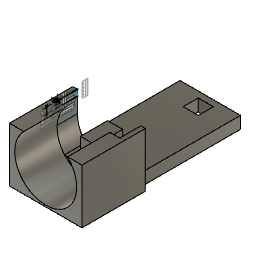
Toggle Box Base v3 (Autodesk Fusion 360 design; units mm, degrees)
Autodesk Fusion 360 part; units mm, degrees
note: some values were not read from the file. Chosen so that the rebuilt part matches the saved one: which face or edge a step refers to; which pieces of a blend or face edit are solid. Set by a fixed rule: which sketch regions a step uses.
sketch "Sketch1" plane through (0, 0, 0) normal (0, 0, 1) x (1, 0, 0)
  line L0 (0, 0) -> (16, 0)
  line L1 (16, 0) -> (16, 29.5)
  line L2 (16, 29.5) -> (0, 29.5)
  line L3 (0, 29.5) -> (0, 0)
  line L4 (-2, -2) -> (18, -2)
  line L5 (18, -2) -> (18, 31.5)
  line L6 (18, 31.5) -> (-2, 31.5)
  line L7 (-2, 31.5) -> (-2, -2)
  dimension "d1" = 16
  dimension "d2" = 29.5
  dimension "d3" = 2
  constraint horizontal L0
  constraint vertical L1
  constraint horizontal L2
  constraint vertical L3
  constraint coincident L0.start L3.end
  measures "d1" distance of L0.start L0.end
  measures "d2" distance of L0.start L2.end
extrude "Extrude1" add sketch "Sketch1" along normal blind 17 makes body 1
sketch "Sketch2" plane through (0, -2, 0) normal (0, -1, 0) x (1, 0, 0)
  line L0 (-2, 0) -> (18, 0)
  line L1 (18, 0) -> (18, 17)
  line L2 (18, 17) -> (-2, 17)
  line L3 (-2, 17) -> (-2, 0)
  line L4 (18, 17) -> (18, 9) construction
  line L5 (18, 9) -> (-2, 9) construction
  line L6 (8, 17) -> (5.5, 17) construction
  line L7 (5.5, 9) -> (2, 7) construction
  line L8 (5.5, 9) -> (10.5, 9) construction
  line L9 (10.5, 9) -> (10.5, 13) construction
  line L10 (10.5, 13) -> (5.5, 13) construction
  line L11 (5.5, 13) -> (5.5, 9) construction
  line L12 (5.5, 13) -> (10.5, 13)
  line L13 (10.5, 13) -> (10.5, 9)
  line L14 (10.5, 9) -> (5.5, 9)
  line L15 (5.5, 9) -> (5.5, 13)
  dimension "d6" = 8
  dimension "d7" = 2.5
  dimension "d8" = 5
  dimension "d9" = 4
  constraint coincident L1.end L2.start
  constraint perpendicular L2 L4
  constraint coincident L3 L5.end
  constraint perpendicular L3 L5
  constraint midpoint L2 L6.start
  constraint coincident L2 L6.end
  constraint coincident L5 L7.start
  constraint horizontal L8
  constraint vertical L9
  constraint horizontal L10
  constraint vertical L11
  constraint horizontal L12
  constraint vertical L13
  constraint horizontal L14
  constraint vertical L15
  measures "d6" distance of L1.end L4.end
  measures "d7" distance of L6.start L6.end
  measures "d8" distance of L7.start L8.end
  measures "d9" distance of L7.start L10.end
extrude "Extrude2" cut sketch "Sketch2" against normal blind 11 contours L12 L13 L14 L15 bodies 1
extrude "Extrude3" add 1 faces at (-1.3333, 19.6667, 0) along direction (0, 0, -1) blind 2 on bodies 1 bodies 1
sketch "Sketch3" plane through (18, 0, 0) normal (1, 0, 0) x (0, 1, 0)
  line L0 (31.5, -2) -> (31.5, 17)
  line L1 (31.5, 17) -> (-2, 17)
  line L2 (-2, 17) -> (-2, -2)
  line L3 (-2, -2) -> (31.5, -2)
  line L4 (-2, -2) -> (31.5, -2)
  line L5 (31.5, -2) -> (31.5, 0)
  line L6 (31.5, 0) -> (-2, 0)
  line L7 (-2, 0) -> (-2, -2)
  dimension "d14" = 2
  constraint horizontal L4
  constraint vertical L5
  constraint horizontal L6
  constraint vertical L7
  constraint coincident L2.end L3.start
  measures "d14" distance of L2.end L6.end
extrude "Extrude4" add sketch "Sketch3" against normal blind 18 contours L0 L2 L3 L4 L5 L6 L7 bodies 1
sketch "Sketch4" plane through (0, 0, 0) normal (0, 0, 1) x (-1, 0, 0)
  line L0 (-16, -29.5) -> (0, -29.5)
  line L1 (0, -29.5) -> (0, 0)
  line L2 (0, 0) -> (-16, 0)
  line L3 (-16, 0) -> (-16, -29.5)
  line L4 (-8, -29.5) -> (-5, -29.5) construction
  line L5 (-5, -29.5) -> (-11, -29.5)
  line L6 (-11, -29.5) -> (-11, -24.5)
  line L7 (-11, -24.5) -> (-5, -24.5)
  line L8 (-5, -24.5) -> (-5, -29.5)
  line L9 (-11, 0) -> (-5, 0)
  line L10 (-5, 0) -> (-5, -5)
  line L11 (-5, -5) -> (-11, -5)
  line L12 (-11, -5) -> (-11, 0)
  dimension "d17" = 3
  dimension "d18" = 6
  dimension "d19" = 5
  dimension "d20" = 6
  dimension "d21" = 5
  constraint midpoint L0 L4.start
  constraint parallel L0 L4
  constraint horizontal L5
  constraint vertical L6
  constraint horizontal L7
  constraint vertical L8
  constraint horizontal L9
  constraint vertical L10
  constraint horizontal L11
  constraint vertical L12
  constraint coincident L2 L9.start
  measures "d17" distance of L4.start L4.end
  measures "d18" distance of L4.end L5.end
  measures "d19" distance of L4.end L7.end
  measures "d20" distance of L9.start L9.end
  measures "d21" distance of L9.start L11.end
extrude "Extrude5" cut sketch "Sketch4" against normal blind 14 contours L0 L5 L6 L7 L8 | L2 L9 L10 L11 L12 bodies 1
extrude "Extrude6" cut 1 faces at (0.3333, 18, -2) along direction (0, 0, 1) blind 2 on bodies 1 bodies 1
extrude "Extrude7" cut 1 faces at (8.8333, -1.3333, 9) along direction (0, 0, -1) blind 25 on bodies 1 bodies 1
extrude "Extrude8" add 1 faces at (-1.3333, 19.6667, 17) along direction (0, 0, 1) blind 1 on bodies 1 bodies 1
sketch "Sketch5" plane through (0, 31.5, 0) normal (0, 1, 0) x (-1, 0, 0)
  line L0 (-18, 0) -> (2, 0)
  line L1 (2, 0) -> (2, 18)
  line L2 (2, 18) -> (-18, 18)
  line L3 (-18, 18) -> (-18, 0)
  line L4 (-18, 18) -> (2, 18)
  line L5 (2, 18) -> (2, 17)
  line L6 (2, 17) -> (-18, 17)
  line L7 (-18, 17) -> (-18, 18)
  dimension "d30" = 1
  constraint horizontal L4
  constraint vertical L5
  constraint horizontal L6
  constraint vertical L7
  constraint coincident L1 L5.end
  constraint coincident L2.end L3.start
  measures "d30" distance of L2.end L6.end
extrude "Extrude9" add sketch "Sketch5" against normal blind 31.5 contours L1 L2 L3 L4 L5 L6 L7 bodies 1
sketch "Sketch6" plane through (0, 0, 18) normal (0, 0, 1) x (-1, 0, 0)
  line L0 (2, -31.5) -> (2, 2)
  line L1 (2, 2) -> (-18, 2)
  line L2 (-18, 2) -> (-18, -31.5)
  line L3 (-18, -31.5) -> (2, -31.5)
  line L4 (2, -31.5) -> (-18, 2) construction
  circle A0 centre (-8, -14.75) radius 6.25
  dimension "d33" = 12.5
  constraint coincident L0.start L3.end
  constraint coincident L1.end L2.start
  constraint midpoint L4 A0.centre
  measures "d33" diameter of A0
extrude "Extrude10" cut sketch "Sketch6" against normal blind 6 contours A0 bodies 1
extrude "Extrude11" add 1 faces at (-1.3333, 19.6667, 0) along direction (0, 0, -1) blind 2 on bodies 1 bodies 1
extrude "Extrude12" cut 1 faces at (7.8443, 27.9942, 18) along direction (0, 0, -1) blind 18 on bodies 1 bodies 1
sketch "Sketch7" plane through (0, 0, 0) normal (0, 0, 1) x (-1, 0, 0)
  line L0 (-5.5, 2) -> (-5.5, 0)
  line L1 (-5.5, 0) -> (0, 0)
  line L2 (0, 0) -> (0, -29.5)
  line L3 (0, -29.5) -> (-16, -29.5)
  line L4 (-16, -29.5) -> (-16, 0)
  line L5 (-16, 0) -> (-10.5, 0)
  line L6 (-10.5, 0) -> (-10.5, 2)
  line L7 (-10.5, 2) -> (-18, 2)
  line L8 (-18, 2) -> (-18, -31.5)
  line L9 (-18, -31.5) -> (2, -31.5)
  line L10 (2, -31.5) -> (2, 2)
  line L11 (2, 2) -> (-5.5, 2)
  line L12 (-5.5, 0) -> (-10.5, 0)
  line L13 (-10.5, 0) -> (-10.5, 2)
  line L14 (-10.5, 2) -> (-5.5, 2)
  line L15 (-5.5, 2) -> (-5.5, 0)
  constraint horizontal L12
  constraint vertical L13
  constraint horizontal L14
  constraint vertical L15
  constraint coincident L6.end L7.start
  constraint coincident L0.end L1.start
extrude "Extrude13" add sketch "Sketch7" along normal blind 8 separate body contours L0 L6 L12 L13 L14 L15 makes body 2
extrude "Extrude14" add 1 faces at (5.5, -1.3333, -0.6667) along direction (1, 0, 0) blind 6 on bodies 1 bodies 1 2
sketch "Sketch8" plane through (0, 0, -2) normal (0, 0, -1) x (1, 0, 0)
  line L0 (0, 0) -> (16, 0)
  line L1 (16, 0) -> (16, -29.5)
  line L2 (16, -29.5) -> (0, -29.5)
  line L3 (0, -29.5) -> (0, 0)
  line L4 (18, 2) -> (-2, 2)
  line L5 (-2, 2) -> (-2, -31.5)
  line L6 (-2, -31.5) -> (18, -31.5)
  line L7 (18, -31.5) -> (18, 2)
extrude "Extrude15" add sketch "Sketch8" against normal blind 2 contours L0 L1 L2 L3 bodies 1
sketch "Sketch9" plane through (0, -2, 0) normal (0, -1, 0) x (1, 0, 0)
  line L0 (-2, -2) -> (18, -2)
  line L1 (18, -2) -> (18, 0)
  line L2 (18, 0) -> (10.5, 0)
  line L3 (10.5, 0) -> (10.5, 8)
  line L4 (10.5, 8) -> (5.5, 8)
  line L5 (5.5, 8) -> (5.5, 0)
  line L6 (5.5, 0) -> (-2, 0)
  line L7 (-2, 0) -> (-2, -2)
  line L8 (5.5, 0) -> (10.5, 0)
  constraint coincident L5.end L6.start
  constraint coincident L2.end L3.start
extrude "Extrude16" add sketch "Sketch9" along normal blind 6 contours L0 L1 L2 L6 L7 L8 bodies 1
sketch "Sketch10" plane through (0, 0, 0) normal (0, 0, 1) x (-1, 0, 0)
  line L0 (-18, 8) -> (-18, -31.5)
  line L1 (-18, -31.5) -> (2, -31.5)
  line L2 (2, -31.5) -> (2, 8)
  line L3 (2, 8) -> (-18, 8)
  line L4 (-10.5, 2) -> (-5.5, 2)
  line L5 (-5.5, 2) -> (-5.5, 0)
  line L6 (-5.5, 0) -> (-10.5, 0)
  line L7 (-10.5, 0) -> (-10.5, 2)
  line L8 (2, 8) -> (-18, 8)
  line L9 (-18, 8) -> (-18, 2)
  line L10 (-18, 2) -> (2, 2)
  line L11 (2, 2) -> (2, 8)
  constraint horizontal L8
  constraint vertical L9
  constraint horizontal L10
  constraint vertical L11
  constraint coincident L0 L9.end
  constraint coincident L2.end L3.start
extrude "Extrude17" add sketch "Sketch10" along normal blind 18 contours L0 L2 L3 L4 L8 L9 L10 L11 bodies 1
sketch "Sketch11" plane through (0, -8, 0) normal (0, -1, 0) x (1, 0, 0)
  line L0 (-2, 18) -> (-2, -2)
  line L1 (-2, -2) -> (18, -2)
  line L2 (18, -2) -> (18, 18)
  line L3 (18, 18) -> (-2, 18)
  line L4 (8, 18) -> (8, 7) construction
  circle A0 centre (8, 7) radius 10
  dimension "d50" = 11
  dimension "d51" = 20
  constraint midpoint L3 L4.start
  constraint perpendicular L3 L4
  constraint coincident L4.end A0.centre
  measures "d50" distance of L4.start L4.end
  measures "d51" diameter of A0
extrude "Extrude18" add 1 faces at (7.1667, -6, 18) along direction (0, 0, -1) blind 22 on bodies 1 bodies 1
extrude "Extrude19" cut sketch "Sketch11" against normal blind 6 contours L1 A0 | L1 A0 bodies 1
extrude "Extrude20" add 2 faces at (0.1449, -8, 15.54) (0.1449, -8, -1.54) along direction (0, -1, 0) blind 15 on bodies 1 bodies 1
extrude "Extrude21" cut 1 faces at (-2, -9, 10.6667) along direction (1, 0, 0) blind 37 on bodies 1 bodies 1
extrude "Extrude22" add 1 faces at (8.8333, -2, 5.3333) along direction (0, -1, 0) blind 7 on bodies 1 bodies 1
sketch "Sketch12" plane through (0, 0, -2) normal (0, 0, -1) x (1, 0, 0)
  line L0 (18, 2) -> (12.3589, 2)
  line L1 (12.3589, 2) -> (12.3589, 9)
  line L2 (12.3589, 9) -> (3.6411, 9)
  line L3 (3.6411, 9) -> (3.6411, 2)
  line L4 (3.6411, 2) -> (-2, 2)
  line L5 (-2, 2) -> (-2, -31.5)
  line L6 (-2, -31.5) -> (18, -31.5)
  line L7 (18, -31.5) -> (18, 2)
  line L8 (12.3589, 2) -> (3.6411, 2)
  constraint coincident L0.end L1.start
  constraint coincident L3.end L4.start
extrude "Extrude23" add sketch "Sketch12" along normal blind 2 contours L1 L2 L3 L8 bodies 1
sketch "Sketch13" plane through (-2, 0, 0) normal (-1, 0, 0) x (0, -1, 0)
  line L0 (23, 7) -> (2, 7)
  line L1 (2, 7) -> (2, 0)
  line L2 (2, 0) -> (-31.5, 0)
  line L3 (-31.5, 0) -> (-31.5, -2)
  line L4 (-31.5, -2) -> (2, -2)
  line L5 (2, -2) -> (2, -4)
  line L6 (2, -4) -> (23, -4)
  line L7 (23, -4) -> (23, 7)
  line L8 (2, 0) -> (2, -2)
  constraint coincident L1.end L2.start
  constraint coincident L4.end L5.start
extrude "Extrude24" add sketch "Sketch13" along normal blind 2 contours L0 L1 L5 L6 L7 L8 bodies 1
sketch "Sketch14" plane through (18, 0, 0) normal (1, 0, 0) x (0, 1, 0)
  line L0 (-2, 7) -> (-23, 7)
  line L1 (-23, 7) -> (-23, -4)
  line L2 (-23, -4) -> (-2, -4)
  line L3 (-2, -4) -> (-2, -2)
  line L4 (-2, -2) -> (31.5, -2)
  line L5 (31.5, -2) -> (31.5, 0)
  line L6 (31.5, 0) -> (-2, 0)
  line L7 (-2, 0) -> (-2, 7)
  line L8 (-2, 0) -> (-2, -2)
  constraint coincident L6.end L7.start
  constraint coincident L3.end L4.start
extrude "Extrude25" add sketch "Sketch14" along normal blind 2 contours L0 L1 L2 L3 L7 L8 bodies 1
extrude "Extrude26" add 2 faces at (19.3333, -9, 7) (-2.6667, -9, 7) along direction (0, 0, 1) blind 7 on bodies 1 bodies 1
move_face "OffsetFaces1" offset -0.5 3 faces at (18, -16, 11.6667) (16.6713, -16, 2.0193) (-2, -9, 9.3333) on bodies 1
sketch "Sketch15" plane through (0, -23, 0) normal (0, -1, 0) x (1, 0, 0)
  arc A0 (-2.5, 7) -> (18.5, 7) centre (8, 7) ccw
  line L0 (-2.5, 7) -> (-2.5, 14)
  line L1 (-2.5, 14) -> (-4, 14)
  line L2 (-4, 14) -> (-4, -4)
  line L3 (-4, -4) -> (20, -4)
  line L4 (20, -4) -> (20, 14)
  line L5 (20, 14) -> (18.5, 14)
  line L6 (18.5, 14) -> (18.5, 7)
  line L7 (8, -3.5) -> (8, -2.25) construction
  line L8 (8, -3.5) -> (8, 6.75) construction
  circle A1 centre (8, 6.75) radius 10.25
  line L9 (20, -4) -> (-4, -4)
  line L10 (-4, -4) -> (-4, 14)
  line L11 (-4, 14) -> (20, 14)
  line L12 (20, 14) -> (20, -4)
  dimension "d71" = 1.25
  dimension "d72" = 10.25
  constraint midpoint A0 L7.start
  constraint perpendicular L3 L7
  constraint parallel L7 L8
  constraint coincident L8.end A1.centre
  constraint coincident L7.start A1
  constraint horizontal L9
  constraint vertical L10
  constraint horizontal L11
  constraint vertical L12
  constraint coincident L1.end L2.start
  constraint coincident L3.end L4.start
  measures "d71" distance of L7.start L7.end
  measures "d72" distance of L7.start L8.end
extrude "Extrude27" add sketch "Sketch15" against normal blind 14 contours A0 L0 A1 L11 | A0 L6 A1 L11 bodies 1
sketch "Sketch16" plane through (-2.5, 0, 0) normal (1, 0, 0) x (0, 1, 0)
  line L0 (-9, 14) -> (-9, 7)
  line L1 (-9, 7) -> (-2, 7)
  line L2 (-2, 7) -> (-2, 14)
  line L3 (-2, 14) -> (-9, 14)
  line L4 (-9, 14) -> (-2, 14)
  line L5 (-2, 14) -> (-2, 12)
  line L6 (-2, 12) -> (-9, 12)
  line L7 (-9, 12) -> (-9, 14)
  dimension "d75" = 2
  constraint horizontal L4
  constraint vertical L5
  constraint horizontal L6
  constraint vertical L7
  constraint coincident L0.start L3.end
  measures "d75" distance of L0.start L6.end
sketch "Sketch17" plane through (0, 0, 0) normal (0, 0, 1) x (-1, 0, 0)
  line L0 (-15.8262, 2) -> (-18, 2)
  line L1 (-18, 2) -> (-18, -31.5)
  line L2 (-18, -31.5) -> (2, -31.5)
  line L3 (2, -31.5) -> (2, 2)
  line L4 (2, 2) -> (-0.1738, 2)
  line L5 (-0.1738, 2) -> (-0.1738, 9)
  line L6 (-0.1738, 9) -> (-0.2864, 9)
  line L7 (-0.2864, 9) -> (-5.5, 9)
  line L8 (-5.5, 9) -> (-5.5, 0)
  line L9 (-5.5, 0) -> (-10.5, 0)
  line L10 (-10.5, 0) -> (-10.5, 9)
  line L11 (-10.5, 9) -> (-15.7136, 9)
  line L12 (-15.7136, 9) -> (-15.8262, 9)
  line L13 (-15.8262, 9) -> (-15.8262, 2)
  line L14 (-8, -31.5) -> (-8, 0) construction
  line L15 (-8, -31.5) -> (-5, -31.5) construction
  line L16 (2, -31.5) -> (2, -28.5) construction
  line L17 (2, -31.5) -> (2, -29.5) construction
  line L18 (2, -29.5) -> (-18, -29.5) construction
  line L19 (-11.03, -29.5) -> (-6.03, -29.5) construction
  line L20 (-6.03, -29.5) -> (-6.03, -24.5) construction
  line L21 (-6.03, -24.5) -> (-11.03, -24.5) construction
  line L22 (-11.03, -24.5) -> (-11.03, -29.5) construction
  line L23 (-8, -29.5) -> (-10.5, -29.5)
  line L24 (-10.5, -29.5) -> (-10.5, 0) construction
  line L25 (2, 0) -> (2, -2) construction
  line L26 (-11.03, -29.5) -> (-6.03, -29.5)
  line L27 (-6.03, -29.5) -> (-6.03, -24.5)
  line L28 (-6.03, -24.5) -> (-11.03, -24.5)
  line L29 (-11.03, -24.5) -> (-11.03, -29.5)
  line L30 (-10.5, -2) -> (-5.5, -2)
  line L31 (-5.5, -2) -> (-5.5, -7)
  line L32 (-5.5, -7) -> (-10.5, -7)
  line L33 (-10.5, -7) -> (-10.5, -2)
  dimension "d76" = 3
  dimension "d77" = 3
  dimension "d78" = 2
  dimension "d79" = 5
  dimension "d80" = 5
  dimension "d81" = 2.5
  dimension "d82" = 2
  dimension "d83" = 5
  dimension "d84" = 5
  dimension "d85" = 5
  constraint midpoint L2 L14.start
  constraint midpoint L9 L14.end
  constraint perpendicular L14 L15
  constraint coincident L2.end L3.start
  constraint perpendicular L2 L16
  constraint perpendicular L2 L17
  constraint coincident L1 L18.end
  constraint perpendicular L1 L18
  constraint horizontal L19
  constraint vertical L20
  constraint horizontal L21
  constraint vertical L22
  constraint coincident L18 L19.start
  constraint midpoint L18 L23.start
  constraint perpendicular L22 L23
  constraint coincident L9.end L10.start
  constraint coincident L3 L25.start
  constraint perpendicular L9 L25
  constraint horizontal L26
  constraint vertical L27
  constraint horizontal L28
  constraint vertical L29
  constraint horizontal L30
  constraint vertical L31
  constraint horizontal L32
  constraint vertical L33
  constraint coincident L24 L30.start
  measures "d76" distance of L14.start L15.end
  measures "d77" distance of L2.end L16.end
  measures "d78" distance of L2.end L17.end
  measures "d79" distance of L19.start L19.end
  measures "d80" distance of L19.start L21.end
  measures "d81" distance of L23.start L23.end
  measures "d82" distance of L25.start L25.end
  measures "d83" distance of L19.start L21.end
  measures "d84" distance of L30.start L30.end
  measures "d85" distance of L30.start L32.end
extrude "Extrude28" cut sketch "Sketch17" against normal blind 25 contours L23 L26 L27 L28 L29 | L30 L31 L32 L33 bodies 1
extrude "Extrude29" add 1 faces at (15.5, 12.1667, -2) along direction (0, 0, -1) blind 2 on bodies 1 bodies 1
